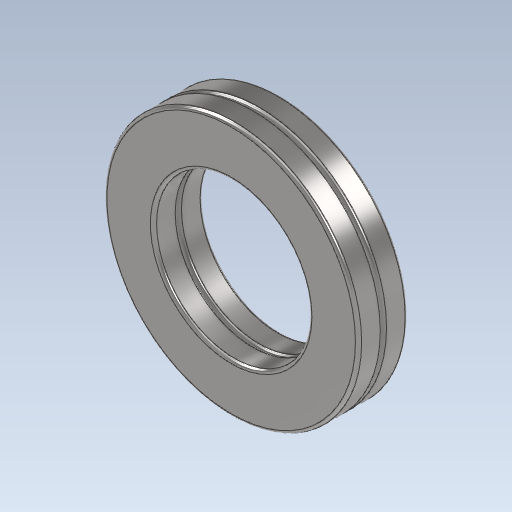
# Autodesk Inventor part: RE2508UUC1
Saved by Autodesk Inventor 2020.4 (Build 244396000, 396)
## iProperties
Part Number: RE2508UUC1
Material: ステンレス鋼 AISI 304
Catalog Web Link: https://jp.misumi-ec.com/vona2/detail/221000091364/?HissuCode=RE2508UUC1
Document SubType Name: Modeling
Designer: Masato Kubotera
Density: 8 g/cm^3
Appearance: 半つや出し
Description: ReadyMade
Mass: 52.5677 g
Surface Area: 33.5275 cm^2
Volume: 6.57097 cm^3
Author: Masato Kubotera
Autodesk Inventor part; units mm, degrees
ref_plane "YZ Plane" through (0, 0, 0) normal (1, 0, 0) x (0, 1, 0)
ref_plane "XZ Plane" through (0, 0, 0) normal (0, 1, 0) x (-1, 0, 0)
ref_plane "XY Plane" through (0, 0, 0) normal (0, 0, 1) x (1, 0, 0)
sketch "スケッチ1" plane through (0, 0, 0) normal (0, 1, 0) x (-1, 0, 0)
  line L0 (-20, 4) -> (-13, 4)
  line L1 (-12.5, 3.5) -> (-12.5, 0.5)
  line L2 (-13, 0) -> (-20, 0) construction
  line L3 (-20.5, 0.5) -> (-20.5, 3.5)
  line L4 (-20.5, 4) -> (-12.5, 0) construction
  line L5 (-12.5, 4) -> (-20.5, 0) construction
  arc A0 (-20, 4) -> (-20.5, 3.5) centre (-20, 3.5) ccw
  arc A1 (-20.5, 0.5) -> (-20, 0) centre (-20, 0.5) ccw
  arc A2 (-13, 0) -> (-12.5, 0.5) centre (-13, 0.5) ccw
  arc A3 (-12.5, 3.5) -> (-13, 4) centre (-13, 3.5) ccw
  line L6 (-20, -4) -> (-13, -4)
  line L7 (-12.5, -3.5) -> (-12.5, -0.5)
  line L8 (-20.5, -0.5) -> (-20.5, -3.5)
  arc A4 (-20, 0) -> (-20.5, -0.5) centre (-20, -0.5) ccw
  arc A5 (-12.5, -0.5) -> (-13, 0) centre (-13, -0.5) ccw
  arc A6 (-13, -4) -> (-12.5, -3.5) centre (-13, -3.5) ccw
  arc A7 (-20.5, -3.5) -> (-20, -4) centre (-20, -3.5) ccw
  line L9 (0, -5.745) -> (0, 5.745) projected
  point P0 (0, 0)
  point P1 (-16.5, 2)
  dimension "d0" = 0.5
  dimension "d1" = 8
  dimension "d2" = 25
  dimension "d3" = 41
  constraints: 18 end point, 16 point on circle, 10 symmetric about line, 9 point on line, 8 centre point, 8 tangent, 3 equal radius, 2 midpoint, 2 parallel, 1 horizontal, 1 perpendicular, 4 other
  measures "d0" radius of A0
  measures "d1" distance of L6.start L0.start
  measures "d2" diameter of L5.start L9
  measures "d3" diameter of L4.start L9
revolve "回転1" add sketch "スケッチ1" angle 360 about axis through (0, 0, -10) along (0, 0, 1)
